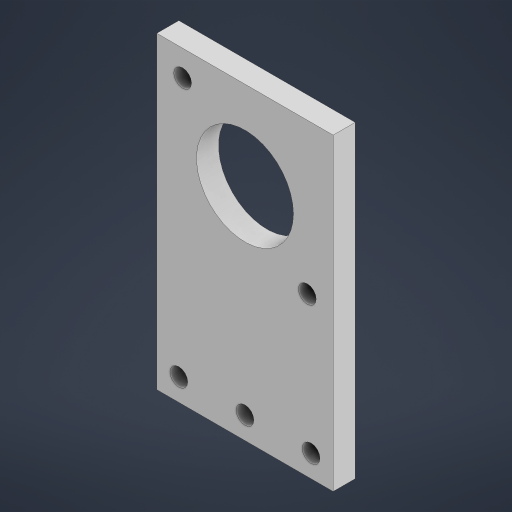
# Autodesk Inventor part: Versaplanetary Mount
Saved by Autodesk Inventor 2023 (Build 270158000, 158)
## iProperties
Created: 2022-05-02
Part Number: Versaplanetary Mount
Material: Generic
Document SubType Name: Modeling
Designer: FizzyApple12
Density: 1 g/cm^3
Appearance: Default
Author: FizzyApple12
Autodesk Inventor part; units mm, degrees
ref_plane "YZ Plane" through (0, 0, 0) normal (1, 0, 0) x (0, 1, 0)
ref_plane "XZ Plane" through (0, 0, 0) normal (0, 1, 0) x (-1, 0, 0)
ref_plane "XY Plane" through (0, 0, 0) normal (0, 0, 1) x (1, 0, 0)
sketch "Sketch1" plane through (0, 0, 0) normal (0, 0, 1) x (1, 0, 0)
  line L0 (0, 0) -> (50.8, 0)
  line L1 (50.8, 0) -> (50.8, -50.8)
  line L2 (50.8, -50.8) -> (0, -50.8)
  line L3 (0, -50.8) -> (0, 0)
  line L4 (0, -50.8) -> (50.8, -50.8)
  line L5 (50.8, -50.8) -> (50.8, -88.9)
  line L6 (50.8, -88.9) -> (0, -88.9)
  line L7 (0, -88.9) -> (0, -50.8)
  line L8 (0, 0) -> (50.8, -50.8) construction
  circle A0 centre (25.4, -25.4) radius 13.97
  point P0 (42.0116, -42.0116)
  dimension "d0" = 50.8
  dimension "d1" = 50.8
  dimension "d2" = 38.1
  dimension "d3" = 27.94
  constraints: 18 end point, 4 parallel, 2 horizontal, 2 perpendicular, 1 centre point, 1 midpoint, 1 point on line
  measures "d0" distance of L1.end L2.end
  measures "d1" distance of L0.end L1.end
  measures "d2" distance of L4.end L5.end
  measures "d3" diameter of A0
extrude "Extrusion1" add sketch "Sketch1" along normal blind 6.35
sketch "Sketch2" plane through (0, 0, 6.35) normal (0, 0, 1) x (1, 0, 0)
  circle A0 centre (25.4, -25.4) radius 13.97 construction
  circle A1 centre (25.4, -25.4) radius 25.4 construction
  line L0 (25.4, -25.4) -> (7.4395, -7.4395) construction
  line L1 (25.4, -25.4) -> (50.8, -25.4) construction
  line L2 (25.4, -25.4) -> (43.3605, -43.3605) construction
  line L3 (25.4, -25.4) -> (50.8, -25.4) construction
  point P0 (0, 0)
  dimension "d6" = 50.8
  dimension "d7" = 25.4
  dimension "d8" = 135
  dimension "d9" = 45
  constraints: 8 end point, 3 coincident, 2 equal length, 2 horizontal, 3 other
  measures "d7" distance of L0.start L0.end
  measures "d8" angle of L1 L0
  measures "d9" angle of L2 L3
hole "Hole1" at (7.4395, -7.4395, 6.35) at (43.3605, -43.3605, 6.35) direction (0, 0, -1) diameter 5.1054 depth 10.795 clearance for "Hex Machine Screw" size "#10" standard "Ansi Unified Screw Threads"
sketch "Sketch3" plane through (0, 0, 6.35) normal (0, 0, 1) x (1, 0, 0)
  line L0 (0, -88.9) -> (50.8, -88.9) construction
  line L1 (50.8, -88.9) -> (50.8, 0) construction
  line L2 (0, -88.9) -> (50.8, -88.9) construction
  line L3 (50.8, -88.9) -> (50.8, -82.55) construction
  line L4 (50.8, -82.55) -> (0, -82.55) construction
  line L5 (0, -82.55) -> (0, -88.9) construction
  line L6 (0, -82.55) -> (25.4, -82.55) construction
  line L7 (25.4, -82.55) -> (50.8, -82.55) construction
  point P0 (0, 0)
  point P1 (6.35, -82.55)
  point P2 (44.45, -82.55)
  dimension "d17" = 6.35
  dimension "d18" = 19.05
  dimension "d19" = 19.05
  constraints: 12 end point, 3 point on line, 2 collinear, 2 parallel, 1 horizontal, 1 midpoint, 1 perpendicular
  measures "d17" distance of L3.end L2.end
  measures "d18" distance of point (6.35, -82.55) L6.end
  measures "d19" distance of point (44.45, -82.55) L6.end
hole "Hole2" at (25.4, -82.55, 6.35) at (6.35, -82.55, 6.35) at (44.45, -82.55, 6.35) direction (0, 0, -1) diameter 5.1054 depth 10.795 clearance for "Hex Machine Screw" size "#10" standard "Ansi Unified Screw Threads"
chamfer "Chamfer1" [suppressed]
body "Solid1"
